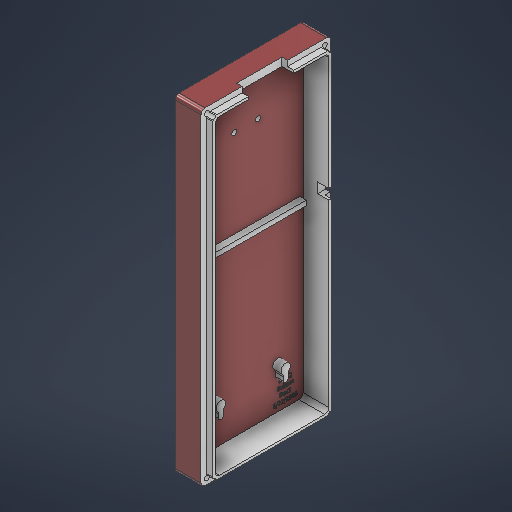
# Autodesk Inventor part: cDAQ_Bottom_Box3
Saved by Autodesk Inventor 2027 (Build 310192000, 192)
## iProperties
Created: 2026-05-08
Part Number: cDAQ_Bottom_Box3
Material: Generic
Document SubType Name: Modeling
Designer: giese
Density: 1 g/cm^3
Appearance: Default
Author: giese
Autodesk Inventor part; units mm, degrees
(part 1 of 2)
ref_plane "YZ Plane" through (0, 0, 0) normal (1, 0, 0) x (0, 1, 0)
ref_plane "XZ Plane" through (0, 0, 0) normal (0, 1, 0) x (-1, 0, 0)
ref_plane "XY Plane" through (0, 0, 0) normal (0, 0, 1) x (1, 0, 0)
sketch "Sketch1" plane through (0, 0, 0) normal (1, 0, 0) x (0, 1, 0)
  line L0 (37.5698, 53.1667) -> (-218.9702, 53.1667)
  line L1 (-218.9702, 53.1667) -> (-218.9702, -48.4333)
  line L2 (-218.9702, -48.4333) -> (37.5698, -48.4333)
  line L3 (37.5698, -48.4333) -> (37.5698, 53.1667)
  point P0 (0, 0)
  dimension "d0" = 101.6
  dimension "d1" = 256.54
  constraints: 8 end point, 2 parallel, 1 horizontal, 1 perpendicular
  measures "d0" distance of L2.end L0.start
  measures "d1" distance of L1.end L2.end
extrude "Extrusion1" add sketch "Sketch1" along normal blind 20.32
sketch "Sketch2" plane through (20.32, 0, 0) normal (1, 0, 0) x (0, 0, -1)
  line L0 (42.0833, 31.2198) -> (-46.8167, 31.2198)
  line L1 (-46.8167, 31.2198) -> (-46.8167, -212.6202)
  line L2 (-46.8167, -212.6202) -> (42.0833, -212.6202)
  line L3 (42.0833, -212.6202) -> (42.0833, 31.2198)
  line L4 (48.4333, 37.5698) -> (-53.1667, 37.5698) projected
  line L5 (-53.1667, 37.5698) -> (-53.1667, -218.9702) projected
  point P0 (0, 0)
  dimension "d4" = 243.84
  dimension "d5" = 88.9
  dimension "d8" = 6.35
  dimension "d21" = 6.35
  constraints: 8 end point, 2 parallel, 1 horizontal, 1 perpendicular
  measures "d4" distance of L2.end L0.start
  measures "d5" distance of L0.start L0.end
  measures "d8" distance between parallel lines of L0 L4
  measures "d21" distance between parallel lines of L5 L1
extrude "Extrusion2" cut sketch "Sketch2" against normal blind 15.24
sketch "Sketch3" plane through (0, 0, 0) normal (-1, 0, 0) x (0, 0, 1)
  circle A0 centre (-6.6909, -5.8642) radius 2
  circle A1 centre (11.8079, -5.8642) radius 2
  circle A2 centre (30.3067, -5.8642) radius 2
  line L0 (-48.4333, -218.9702) -> (-48.4333, 37.5698) projected
  line L1 (-48.4333, 37.5698) -> (53.1667, 37.5698) projected
  line L2 (53.1667, 37.5698) -> (53.1667, -218.9702) projected
  line L3 (46.8167, 31.2198) -> (-42.0833, 31.2198) projected
  point P0 (0, 0)
  point P1 (-0.896, -23.7433)
  point P2 (-45.1848, 27.0137)
  dimension "d9" = 18.4988
  dimension "d10" = 4
  dimension "d11" = 4
  dimension "d12" = 18.4988
  dimension "d13" = 36.9976
  dimension "d18" = 22.86
  dimension "d22" = 4
  dimension "d58" = 43.434
  constraints: 3 centre point
  measures "d9" distance of A0.centre A1.centre
  measures "d10" diameter of A1
  measures "d11" diameter of A2
  measures "d12" distance of A1.centre A2.centre
  measures "d13" distance of A0.centre A2.centre
  measures "d18" distance from line of L2 A2.centre
  measures "d22" diameter of A0
  measures "d58" distance from line of L1 A2.centre
extrude "Extrusion3" cut sketch "Sketch3" against normal blind 5.08
sketch "Sketch5" plane through (0, -218.9702, -48.4333) normal (0, 0, -1) x (-1, 0, 0)
  line L0 (-27.2034, 150.2918) -> (-16.51, 150.2918)
  line L1 (-16.51, 150.2918) -> (-16.51, 158.2918)
  line L2 (-16.51, 158.2918) -> (-27.2034, 158.2918)
  line L3 (-27.2034, 158.2918) -> (-27.2034, 150.2918)
  line L4 (0, 256.54) -> (-20.32, 256.54) projected
  line L5 (0, 0) -> (0, 256.54) projected
  line L6 (-20.32, 0) -> (-20.32, 256.54) projected
  point P0 (0, 218.9702)
  point P1 (-21.8567, 158.2918)
  point P2 (-21.8567, 150.2918)
  dimension "d28" = 10.6934
  dimension "d30" = 8
  dimension "d31" = 16.51
  dimension "d34" = 106.2482
  dimension "d215" = 6.8834
  constraints: 8 end point, 2 midpoint, 2 parallel, 1 horizontal, 1 perpendicular
  measures "d28" distance between parallel lines of L1 L3
  measures "d30" distance of point (-21.857, 158.292) point (-21.857, 150.292)
  measures "d31" distance between parallel lines of L5 L1
  measures "d34" distance between parallel lines of L4 L0
  measures "d215" distance between parallel lines of L6 L3
extrude "Extrusion4" cut sketch "Sketch5" against normal blind 24.13
sketch "Sketch6" plane through (0, -218.9702, -48.4333) normal (0, -1, 0) x (1, 0, 0)
  line L0 (24.08, 45.1284) -> (16.08, 45.1284)
  line L1 (16.08, 45.1284) -> (16.08, 35.1284)
  line L2 (16.08, 35.1284) -> (24.08, 35.1284)
  line L3 (0, 101.6) -> (0, 0) projected
  line L4 (25.82, 43.1283) -> (25.82, 37.1284)
  line L5 (24.08, 45.1284) -> (25.82, 43.1283)
  line L6 (25.82, 37.1284) -> (24.08, 35.1284)
  line L7 (0, 0) -> (20.32, 0) projected
  line L8 (20.32, 95.25) -> (20.32, 6.35) projected
  line L9 (20.32, 41.9134) -> (20.32, 37.4697)
  point P0 (0, 48.4333)
  point P1 (20.08, 45.1284)
  point P2 (20.08, 35.1284)
  point P3 (16.08, 40.1284)
  dimension "d35" = 10
  dimension "d39" = 6
  dimension "d48" = 45.1284
  dimension "d220" = 16.08
  dimension "d221" = 0
  dimension "d222" = 8
  dimension "d223" = 2
  dimension "d224" = 2
  dimension "d225" = 5.5
  dimension "d226" = 4.24
  dimension "d227" = 1.74
  constraints: 14 end point, 3 midpoint, 2 point on line, 1 horizontal, 1 parallel, 1 perpendicular, 1 vertical
  measures "d35" distance of point (20.08, 45.128) point (20.08, 35.128)
  measures "d39" distance of L4.start L4.end
  measures "d48" distance between parallel lines of L7 L0
  measures "d220" distance from line of L3 point (16.08, 40.128)
  measures "d221" horizontal distance of L0.start L2.end
  measures "d222" distance of L1.end L2.end
  measures "d223" vertical distance of L4.end L2.end
  measures "d224" vertical distance of L0.start L4.start
  measures "d225" distance between parallel lines of L4 L8
  measures "d226" distance between parallel lines of L1 L8
  measures "d227" distance from line of L2.end L4
extrude "Extrusion5" cut sketch "Sketch6" against normal blind 3.81
sketch "Sketch7" plane through (0, 37.5698, 53.1667) normal (0, 1, 0) x (1, 0, 0)
  line L0 (31.0134, 67.818) -> (16.002, 67.818)
  line L1 (16.002, 67.818) -> (16.002, 32.258)
  line L2 (16.002, 32.258) -> (31.0134, 32.258)
  line L3 (31.0134, 32.258) -> (31.0134, 67.818)
  line L4 (0, 0) -> (20.32, 0) projected
  line L5 (0, 101.6) -> (0, 0) projected
  line L6 (20.32, 101.6) -> (20.32, 0) projected
  point P0 (0, 53.1667)
  point P1 (20.32, 67.818)
  point P2 (20.32, 32.258)
  dimension "d51" = 35.56
  dimension "d52" = 32.258
  dimension "d55" = 16.002
  dimension "d56" = 15.0114
  dimension "d57" = 10.6934
  constraints: 8 end point, 2 parallel, 1 horizontal, 1 perpendicular
  measures "d51" distance of L2.end L0.start
  measures "d52" distance between parallel lines of L4 L2
  measures "d55" distance between parallel lines of L5 L1
  measures "d56" distance between parallel lines of L3 L1
  measures "d57" distance between parallel lines of L6 L3
extrude "Extrusion6" cut sketch "Sketch7" against normal blind 7.62
fillet "Fillet1" radius 3.175 4 edges at (10.16, 37.5698, -48.4333) (10.16, 37.5698, 53.1667) (10.16, -218.9702, -48.4333) (10.16, -218.9702, 53.1667)
sketch "Sketch8" plane through (0, 0, 0) normal (-1, 0, 0) x (0, 0, 1)
  line L0 (-8.4625, -9.3948) -> (-4.9319, -9.3948)
  line L1 (-8.4625, -2.3336) -> (-4.9319, -2.3336)
  line L2 (-8.4625, -9.3948) -> (-10.5009, -5.8642)
  line L3 (-8.4625, -2.3336) -> (-10.5009, -5.8642)
  line L4 (-4.9319, -9.3948) -> (-2.8936, -5.8642)
  line L5 (-4.9319, -2.3336) -> (-2.8936, -5.8642)
  circle A0 centre (-6.6909, -5.8642) radius 2 projected
  line L6 (10.0363, -9.3948) -> (13.5669, -9.3948)
  line L7 (10.0363, -2.3336) -> (13.5669, -2.3336)
  line L8 (10.0363, -9.3948) -> (7.9979, -5.8642)
  line L9 (10.0363, -2.3336) -> (7.9979, -5.8642)
  line L10 (13.5669, -9.3948) -> (15.6053, -5.8642)
  line L11 (13.5669, -2.3336) -> (15.6053, -5.8642)
  circle A1 centre (11.8079, -5.8642) radius 2 projected
  line L12 (28.5351, -9.3948) -> (26.4967, -5.8642)
  line L13 (28.5351, -2.3336) -> (26.4967, -5.8642)
  line L14 (28.5351, -9.3948) -> (32.0657, -9.3948)
  line L15 (28.5351, -2.3336) -> (32.0657, -2.3336)
  line L16 (32.0657, -9.3948) -> (34.1041, -5.8642)
  line L17 (32.0657, -2.3336) -> (34.1041, -5.8642)
  circle A2 centre (30.3067, -5.8642) radius 2 projected
  point P0 (-6.6972, -9.3948)
  point P1 (11.8016, -9.3948)
  point P2 (30.3004, -9.3948)
  point P3 (-10.5009, -5.8642)
  point P4 (-2.8936, -5.8642)
  point P5 (15.6053, -5.8642)
  point P6 (7.9979, -5.8642)
  point P7 (34.1041, -5.8642)
  dimension "d60" = 7.0612
  dimension "d61" = 120
  dimension "d62" = 120
  dimension "d63" = 120
  dimension "d64" = 120
  dimension "d65" = 3.5306
  dimension "d66" = 3.5306
  dimension "d67" = 3.5306
  dimension "d68" = 3.5306
  dimension "d69" = 3.5306
  dimension "d70" = 3.5306
  dimension "d71" = 0
  dimension "d72" = 7.6074
  dimension "d73" = 3.81
  dimension "d74" = 0
  dimension "d75" = 7.0612
  dimension "d76" = 120
  dimension "d77" = 120
  dimension "d78" = 120
  dimension "d79" = 120
  dimension "d80" = 3.5306
  dimension "d81" = 3.5306
  dimension "d82" = 3.5306
  dimension "d83" = 3.5306
  dimension "d84" = 3.5306
  dimension "d85" = 3.5306
  dimension "d86" = 0
  dimension "d87" = 7.6074
  dimension "d91" = 0
  dimension "d92" = 3.81
  dimension "d93" = 7.0612
  dimension "d94" = 120
  dimension "d95" = 120
  dimension "d96" = 120
  dimension "d97" = 120
  dimension "d98" = 3.5306
  dimension "d99" = 3.5306
  dimension "d100" = 3.5306
  dimension "d101" = 3.5306
  dimension "d102" = 3.5306
  dimension "d103" = 3.5306
  dimension "d104" = 0
  dimension "d105" = 7.6074
  dimension "d108" = 0
  dimension "d109" = 3.81
  constraints: 36 end point, 6 horizontal, 3 midpoint
  measures "d60" distance from line of point (-6.697, -9.395) L1
  measures "d61" angle of L0 L2
  measures "d62" angle of L1 L3
  measures "d63" angle of L4 L0
  measures "d64" angle of L5 L1
  measures "d65" distance of L0.start L0.end
  measures "d66" distance of L1.start L1.end
  measures "d67" vertical distance of L1.start L3.end
  measures "d68" vertical distance of L0.start L2.end
  measures "d69" vertical distance of L1.end L5.end
  measures "d70" vertical distance of L0.end L4.end
  measures "d71" horizontal distance of L0.start L1.start
  measures "d72" distance of L4.end L2.end
  measures "d73" distance of A0.centre L2.end
  measures "d74" vertical distance of A0.centre L4.end
  measures "d75" distance from line of point (11.802, -9.395) L7
  measures "d76" angle of L6 L8
  measures "d77" angle of L7 L9
  measures "d78" angle of L10 L6
  measures "d79" angle of L11 L7
  measures "d80" distance of L8.start L6.end
  measures "d81" distance of L9.start L7.end
  measures "d82" vertical distance of L9.start L9.end
  measures "d83" vertical distance of L8.start L8.end
  measures "d84" vertical distance of L7.end L11.end
  measures "d85" vertical distance of L6.end L10.end
  measures "d86" horizontal distance of L8.start L9.start
  measures "d87" distance of L10.end L8.end
  measures "d91" vertical distance of A1.centre L8.end
  measures "d92" distance of A1.centre L8.end
  measures "d93" distance from line of point (30.3, -9.395) L15
  measures "d94" angle of L14 L12
  measures "d95" angle of L15 L13
  measures "d96" angle of L16 L14
  measures "d97" angle of L17 L15
  measures "d98" distance of L12.start L16.start
  measures "d99" distance of L15.start L15.end
  measures "d100" vertical distance of L15.start L13.end
  measures "d101" vertical distance of L12.start L12.end
  measures "d102" vertical distance of L15.end L17.end
  measures "d103" vertical distance of L16.start L16.end
  measures "d104" horizontal distance of L12.start L15.start
  measures "d105" distance of L16.end L12.end
  measures "d108" vertical distance of A2.centre L12.end
  measures "d109" distance of A2.centre L12.end
extrude "Extrusion7" cut sketch "Sketch8" against normal blind 0.9525 contours L2 L3 L1 L5 L4 L0 | A0 | L8 L9 L7 L11 L10 L6 | A1 | L12 L13 L15 L17 L16 L14 | A2
sketch "Sketch9" plane through (5.08, 0, 0) normal (1, 0, 0) x (0, 0, -1)
  arc A0 (24.8089, -182.3284) -> (19.3527, -182.3284) centre (22.0808, -179.8542) ccw
  line L0 (45.2583, 37.5698) -> (14.6513, 37.5698) projected
  line L1 (42.0833, 31.2198) -> (42.0833, -212.6202) projected
  arc A1 (20.1758, -187.4742) -> (23.9858, -187.4742) centre (22.0808, -187.4742) ccw
  line L2 (23.9858, -187.4742) -> (23.9858, -184.4614)
  line L3 (20.1758, -187.4742) -> (20.1758, -184.4614)
  arc A2 (24.8089, -182.3284) -> (23.9858, -184.4614) centre (27.1608, -184.4614) ccw
  arc A3 (20.1758, -184.4614) -> (19.3527, -182.3284) centre (17.0008, -184.4614) ccw
  arc A4 (-25.9911, -182.3284) -> (-31.4473, -182.3285) centre (-28.7192, -179.8542) ccw
  arc A5 (-30.6242, -187.4606) -> (-26.8142, -187.4742) centre (-28.7192, -187.4742) ccw
  line L4 (-26.8142, -187.4742) -> (-26.8142, -184.4614)
  line L5 (-30.6242, -187.4606) -> (-30.6242, -184.4614)
  arc A6 (-25.9911, -182.3284) -> (-26.8142, -184.4614) centre (-23.6392, -184.4614) ccw
  arc A7 (-30.6242, -184.4614) -> (-31.4473, -182.3285) centre (-33.7992, -184.4614) ccw
  line L6 (-20.9087, 37.5698) -> (-49.9917, 37.5698) projected
  line L7 (-46.8167, -212.6202) -> (-46.8167, 31.2198) projected
  point P0 (0, 0)
  point P1 (23.9858, -183.0063)
  point P2 (20.1758, -183.0063)
  point P3 (-26.8142, -183.0063)
  point P4 (-30.6242, -183.0063)
  dimension "d112" = 217.424
  dimension "d114" = 7.366
  dimension "d116" = 3.81
  dimension "d117" = 225.044
  dimension "d118" = 3.175
  dimension "d119" = 7.366
  dimension "d120" = 3.81
  dimension "d121" = 3.175
  dimension "d122" = 217.424
  dimension "d123" = 225.044
  dimension "d125" = 0
  dimension "d128" = 50.8
  dimension "d129" = 20.0025
  dimension "d130" = 0
  constraints: 20 point on circle, 8 centre point, 8 end point, 8 tangent, 4 point on line, 2 equal radius, 2 parallel, 2 vertical
  measures "d112" distance from line of L0 A0.centre
  measures "d114" diameter of A0
  measures "d116" diameter of A1
  measures "d117" distance from line of L0 A1.centre
  measures "d118" radius of A2
  measures "d119" diameter of A4
  measures "d120" diameter of A5
  measures "d121" radius of A6
  measures "d122" distance from line of A4.centre L6
  measures "d123" distance from line of L6 A5.centre
  measures "d125" horizontal distance of A5.centre A4.centre
  measures "d128" distance of A5.centre A1.centre
  measures "d129" distance from line of L1 A0.centre
  measures "d130" horizontal distance of A0.centre A1.centre
extrude "Extrusion8" add sketch "Sketch9" along normal blind 6.4008
sketch "Sketch10" plane through (20.32, 0, 0) normal (1, 0, 0) x (0, 0, -1)
  line L0 (-46.8167, 31.2198) -> (42.0833, 31.2198) projected
  line L1 (-46.8167, 31.2198) -> (42.0833, 31.2198)
  line L2 (42.0833, 33.2264) -> (-46.8167, 33.2264)
  line L3 (-46.8167, 33.2264) -> (-48.8233, 33.2264)
  line L4 (-48.8233, 33.2264) -> (-48.8233, -214.6268)
  line L5 (-48.8233, -214.6268) -> (44.0899, -214.6268)
  line L6 (44.0899, -214.6268) -> (44.0899, 33.2264)
  line L7 (44.0899, 33.2264) -> (41.9392, 33.2264)
  line L8 (42.0833, 31.2198) -> (42.0833, -212.6202) projected
  line L9 (-46.8167, -212.6202) -> (-46.8167, 31.2198) projected
  line L10 (42.0833, -212.6202) -> (-46.8167, -212.6202) projected
  line L11 (45.2583, 37.5698) -> (14.6513, 37.5698) projected
  dimension "d202" = 2.0066
  dimension "d203" = 2.0066
  dimension "d204" = 2.0066
  dimension "d205" = 2.0066
  dimension "d208" = 4.3434
  constraints: 14 end point, 3 perpendicular, 3 point on line, 1 collinear, 1 horizontal
  measures "d202" distance between parallel lines of L0 L2
  measures "d203" distance between parallel lines of L6 L8
  measures "d204" distance between parallel lines of L4 L9
  measures "d205" distance between parallel lines of L5 L10
  measures "d208" distance between parallel lines of L11 L2
extrude "Extrusion9" add sketch "Sketch10" along normal blind 5
fillet "Fillet2" radius 3.175 8 edges at (15.2, 31.2198, -42.0833) (15.2, 31.2198, 46.8167) (15.2, -212.6202, 46.8167) (15.2, -212.6202, -42.0833) (22.82, 33.2264, -44.0899) (22.82, 33.2264, 48.8233) (22.82, -214.6268, -44.0899) (22.82, -214.6268, 48.8233)
sketch "Sketch13" plane through (25.32, 0, 0) normal (1, 0, 0) x (0, 0, -1)
  arc A0 (44.0833, 30.0448) -> (40.9083, 33.2198) centre (40.9083, 30.0448) ccw projected
  arc A1 (-45.6417, 33.2198) -> (-48.8167, 30.0448) centre (-45.6417, 30.0448) ccw projected
  arc A2 (40.9083, -212.0802) -> (44.0833, -208.9052) centre (40.9083, -208.9052) ccw projected
  arc A3 (-48.8167, -208.9052) -> (-45.6417, -212.0802) centre (-45.6417, -208.9052) ccw projected
  line L0 (-20.9087, 37.5698) -> (-49.9917, 37.5698) projected
  line L1 (-53.1667, 34.3948) -> (-53.1667, -215.7952) projected
  line L2 (-49.9917, -218.9702) -> (45.2583, -218.9702) projected
  arc A4 (-48.8167, -208.9052) -> (-45.6417, -212.0802) centre (-45.6417, -208.9052) ccw projected
  circle A5 centre (-48.5947, -214.3982) radius 1.9939
  circle A6 centre (43.8613, -214.3982) radius 1.9939
  line L3 (48.4333, -215.7952) -> (48.4333, 34.3948) projected
  circle A7 centre (43.8613, 32.9978) radius 1.9939
  line L4 (45.2583, 37.5698) -> (14.6513, 37.5698) projected
  circle A8 centre (-48.5947, 32.9978) radius 1.9939
  point P0 (0, 0)
  point P1 (-47.8868, 32.2898)
  point P2 (-47.8868, -211.1503)
  point P3 (-47.8868, -211.1503)
  dimension "d178" = 4.572
  dimension "d179" = 4.572
  dimension "d180" = 3.9878
  dimension "d181" = 4.572
  dimension "d182" = 4.572
  dimension "d183" = 3.9878
  dimension "d184" = 3.9878
  dimension "d185" = 4.572
  dimension "d186" = 4.572
  dimension "d187" = 3.9878
  dimension "d188" = 4.572
  dimension "d189" = 4.572
  constraints: 4 centre point, 3 point on circle
  measures "d178" distance from line of L1 A5.centre
  measures "d179" distance from line of L2 A5.centre
  measures "d180" diameter of A5
  measures "d181" distance from line of L2 A6.centre
  measures "d182" distance from line of L3 A6.centre
  measures "d183" diameter of A6
  measures "d184" diameter of A7
  measures "d185" distance from line of L3 A7.centre
  measures "d186" distance from line of L4 A7.centre
  measures "d187" diameter of A8
  measures "d188" distance from line of L0 A8.centre
  measures "d189" distance from line of L1 A8.centre
extrude "Extrusion11" cut sketch "Sketch13" against normal blind 25.4
sketch "Sketch14" plane through (5.08, 0, 0) normal (1, 0, 0) x (0, 0, -1)
  line L0 (18.5513, -190.7882) -> (37.7681, -190.7882) construction
  line L1 (37.7681, -190.7882) -> (37.7681, -199.5809) construction
  line L2 (37.7681, -199.5809) -> (18.5513, -199.5809) construction
  line L3 (18.5513, -199.5809) -> (18.5513, -190.7882) construction
  spline S0 degree 2 poles (24.2188, -193.9523) (23.9817, -193.9523) (23.5889, -193.8066) (23.4481, -193.6584) knots 0 0 0 1 2 2 2
  spline S1 degree 2 poles (23.4481, -193.6584) (23.3073, -193.5127) (23.1517, -193.0631) (23.1517, -192.7618) knots 0 0 0 1 2 2 2
  spline S2 degree 2 poles (23.1517, -192.7618) (23.1517, -192.4604) (23.3123, -192.0208) (23.4481, -191.8726) knots 0 0 0 1 2 2 2
  spline S3 degree 2 poles (23.4481, -191.8726) (23.584, -191.7219) (23.9866, -191.5614) (24.2188, -191.5614) knots 0 0 0 1 2 2 2
  spline S4 degree 2 poles (24.2188, -191.5614) (24.4065, -191.5614) (24.7572, -191.6676) (24.8931, -191.7367) knots 0 0 0 1 2 2 2
  line L4 (24.8931, -191.7367) -> (24.8931, -192.169)
  line L5 (24.8931, -192.169) -> (24.8709, -192.169)
  spline S5 degree 2 poles (24.8709, -192.169) (24.8289, -192.1344) (24.7004, -192.0455) (24.609, -191.9985) knots 0 0 0 1 2 2 2
  spline S6 degree 2 poles (24.609, -191.9985) (24.5275, -191.959) (24.3102, -191.8973) (24.2114, -191.8973) knots 0 0 0 1 2 2 2
  spline S7 degree 2 poles (24.2114, -191.8973) (23.9125, -191.8973) (23.5494, -192.3493) (23.5494, -192.7618) knots 0 0 0 1 2 2 2
  spline S8 degree 2 poles (23.5494, -192.7618) (23.5494, -193.1644) (23.9002, -193.6164) (24.2114, -193.6164) knots 0 0 0 1 2 2 2
  spline S9 degree 2 poles (24.2114, -193.6164) (24.3991, -193.6164) (24.74, -193.4608) (24.8709, -193.3398) knots 0 0 0 1 2 2 2
  line L6 (24.8709, -193.3398) -> (24.8931, -193.3398)
  line L7 (24.8931, -193.3398) -> (24.8931, -193.772)
  spline S10 degree 2 poles (24.8931, -193.772) (24.8363, -193.7992) (24.6634, -193.8758) (24.5942, -193.8931) knots 0 0 0 1 2 2 2
  spline S11 degree 2 poles (24.5942, -193.8931) (24.4954, -193.9227) (24.3398, -193.9523) (24.2188, -193.9523) knots 0 0 0 1 2 2 2
  spline S12 degree 2 poles (27.6768, -192.3789) (27.6768, -192.7964) (27.3384, -193.4682) (27.0544, -193.6559) knots 0 0 0 1 2 2 2
  spline S13 degree 2 poles (27.0544, -193.6559) (26.8222, -193.8017) (26.3455, -193.9005) (25.975, -193.9005) knots 0 0 0 1 2 2 2
  line L8 (25.975, -193.9005) -> (25.2735, -193.9005)
  line L9 (25.2735, -193.9005) -> (25.2735, -190.8525)
  line L10 (25.2735, -190.8525) -> (25.9676, -190.8525)
  spline S14 degree 2 poles (25.9676, -190.8525) (26.3973, -190.8525) (26.8864, -190.9809) (27.0593, -191.0945) knots 0 0 0 1 2 2 2
  spline S15 degree 2 poles (27.0593, -191.0945) (27.3532, -191.2897) (27.6768, -191.9343) (27.6768, -192.3789) knots 0 0 0 1 2 2 2
  spline S16 degree 2 poles (27.2544, -192.374) (27.2544, -192.0233) (27.0223, -191.5268) (26.7925, -191.386) knots 0 0 0 1 2 2 2
  spline S17 degree 2 poles (26.7925, -191.386) (26.6295, -191.2897) (26.2615, -191.2032) (25.9873, -191.2032) knots 0 0 0 1 2 2 2
  line L11 (25.9873, -191.2032) -> (25.6786, -191.2032)
  line L12 (25.6786, -191.2032) -> (25.6786, -193.5497)
  line L13 (25.6786, -193.5497) -> (25.9873, -193.5497)
  spline S18 degree 2 poles (25.9873, -193.5497) (26.2565, -193.5497) (26.6641, -193.4633) (26.8296, -193.3472) knots 0 0 0 1 2 2 2
  spline S19 degree 2 poles (26.8296, -193.3472) (27.042, -193.2039) (27.2544, -192.7297) (27.2544, -192.374) knots 0 0 0 1 2 2 2
  line L14 (27.788, -193.9005) -> (28.8155, -190.8525)
  line L15 (28.8155, -190.8525) -> (29.3144, -190.8525)
  line L16 (29.3144, -190.8525) -> (30.342, -193.9005)
  line L17 (30.342, -193.9005) -> (29.9146, -193.9005)
  line L18 (29.9146, -193.9005) -> (29.638, -193.0483)
  line L19 (29.638, -193.0483) -> (28.4746, -193.0483)
  line L20 (28.4746, -193.0483) -> (28.198, -193.9005)
  line L21 (28.198, -193.9005) -> (27.788, -193.9005)
  line L22 (29.5268, -192.7025) -> (29.0551, -191.2674)
  line L23 (29.0551, -191.2674) -> (28.5858, -192.7025)
  line L24 (28.5858, -192.7025) -> (29.5268, -192.7025)
  spline S20 degree 2 poles (33.1627, -194.6464) (33.0516, -194.6736) (32.8095, -194.7032) (32.6885, -194.7032) knots 0 0 0 1 2 2 2
  spline S21 degree 2 poles (32.6885, -194.7032) (32.3451, -194.7032) (31.9178, -194.3204) (31.8981, -193.9647) knots 0 0 0 1 2 2 2
  spline S22 degree 2 poles (31.8981, -193.9647) (31.8709, -193.9647) (31.824, -193.9647) (31.8042, -193.9647) knots 0 0 0 1 2 2 2
  spline S23 degree 2 poles (31.8042, -193.9647) (31.4955, -193.9647) (30.999, -193.7547) (30.8211, -193.5497) knots 0 0 0 1 2 2 2
  spline S24 degree 2 poles (30.8211, -193.5497) (30.6458, -193.3472) (30.458, -192.7544) (30.458, -192.3789) knots 0 0 0 1 2 2 2
  spline S25 degree 2 poles (30.458, -192.3789) (30.458, -191.9936) (30.6482, -191.4107) (30.8236, -191.2032) knots 0 0 0 1 2 2 2
  spline S26 degree 2 poles (30.8236, -191.2032) (31.0014, -190.9982) (31.4979, -190.7882) (31.8042, -190.7882) knots 0 0 0 1 2 2 2
  spline S27 degree 2 poles (31.8042, -190.7882) (32.1154, -190.7882) (32.6144, -191.0056) (32.7873, -191.2032) knots 0 0 0 1 2 2 2
  spline S28 degree 2 poles (32.7873, -191.2032) (32.9602, -191.4033) (33.1528, -191.9985) (33.1528, -192.3789) knots 0 0 0 1 2 2 2
  spline S29 degree 2 poles (33.1528, -192.3789) (33.1528, -192.9717) (32.6909, -193.7424) (32.2883, -193.8782) knots 0 0 0 1 2 2 2
  spline S30 degree 2 poles (32.2883, -193.8782) (32.2982, -193.9919) (32.3575, -194.1746) (32.4044, -194.2265) knots 0 0 0 1 2 2 2
  spline S31 degree 2 poles (32.4044, -194.2265) (32.4612, -194.2907) (32.6168, -194.35) (32.7552, -194.35) knots 0 0 0 1 2 2 2
  spline S32 degree 2 poles (32.7552, -194.35) (32.8367, -194.35) (33.059, -194.2981) (33.1084, -194.2784) knots 0 0 0 1 2 2 2
  line L25 (33.1084, -194.2784) -> (33.1627, -194.2784)
  line L26 (33.1627, -194.2784) -> (33.1627, -194.6464)
  spline S33 degree 2 poles (32.7305, -192.3789) (32.7305, -192.0751) (32.5995, -191.6083) (32.481, -191.4551) knots 0 0 0 1 2 2 2
  spline S34 degree 2 poles (32.481, -191.4551) (32.36, -191.2971) (32.0191, -191.139) (31.8067, -191.139) knots 0 0 0 1 2 2 2
  spline S35 degree 2 poles (31.8067, -191.139) (31.5868, -191.139) (31.2559, -191.2921) (31.1299, -191.4551) knots 0 0 0 1 2 2 2
  spline S36 degree 2 poles (31.1299, -191.4551) (31.0089, -191.6108) (30.8804, -192.0825) (30.8804, -192.3789) knots 0 0 0 1 2 2 2
  spline S37 degree 2 poles (30.8804, -192.3789) (30.8804, -192.9791) (31.3843, -193.6189) (31.8067, -193.6189) knots 0 0 0 1 2 2 2
  spline S38 degree 2 poles (31.8067, -193.6189) (32.229, -193.6189) (32.7305, -192.9791) (32.7305, -192.3789) knots 0 0 0 1 2 2 2
  spline S39 degree 2 poles (23.8631, -197.9828) (23.8631, -198.21) (23.6902, -198.5583) (23.5469, -198.6719) knots 0 0 0 1 2 2 2
  spline S40 degree 2 poles (23.5469, -198.6719) (23.374, -198.8053) (22.9813, -198.9189) (22.6701, -198.9189) knots 0 0 0 1 2 2 2
  line L27 (22.6701, -198.9189) -> (21.7957, -198.9189)
  line L28 (21.7957, -198.9189) -> (21.7957, -195.8709)
  line L29 (21.7957, -195.8709) -> (22.6034, -195.8709)
  spline S41 degree 2 poles (22.6034, -195.8709) (22.9294, -195.8709) (23.2555, -195.9129) (23.4037, -195.9944) knots 0 0 0 1 2 2 2
  spline S42 degree 2 poles (23.4037, -195.9944) (23.5692, -196.0809) (23.7198, -196.3649) (23.7198, -196.5576) knots 0 0 0 1 2 2 2
  spline S43 degree 2 poles (23.7198, -196.5576) (23.7198, -196.7725) (23.4926, -197.1133) (23.2925, -197.2097) knots 0 0 0 1 2 2 2
  line L30 (23.2925, -197.2097) -> (23.2925, -197.2245)
  spline S44 degree 2 poles (23.2925, -197.2245) (23.5642, -197.2986) (23.8631, -197.6913) (23.8631, -197.9828) knots 0 0 0 1 2 2 2
  spline S45 degree 2 poles (23.4407, -198.0001) (23.4407, -197.8272) (23.3419, -197.6049) (23.1937, -197.5258) knots 0 0 0 1 2 2 2
  spline S46 degree 2 poles (23.1937, -197.5258) (23.0974, -197.4764) (22.8702, -197.4468) (22.6602, -197.4468) knots 0 0 0 1 2 2 2
  line L31 (22.6602, -197.4468) -> (22.2008, -197.4468)
  line L32 (22.2008, -197.4468) -> (22.2008, -198.5731)
  line L33 (22.2008, -198.5731) -> (22.5293, -198.5731)
  spline S47 degree 2 poles (22.5293, -198.5731) (22.7961, -198.5731) (23.1023, -198.5237) (23.2209, -198.4447) knots 0 0 0 1 2 2 2
  spline S48 degree 2 poles (23.2209, -198.4447) (23.3345, -198.3632) (23.4407, -198.1606) (23.4407, -198.0001) knots 0 0 0 1 2 2 2
  spline S49 degree 2 poles (23.2975, -196.6144) (23.2975, -196.5057) (23.2234, -196.3427) (23.1419, -196.2958) knots 0 0 0 1 2 2 2
  spline S50 degree 2 poles (23.1419, -196.2958) (23.0431, -196.2414) (22.8035, -196.2167) (22.5886, -196.2167) knots 0 0 0 1 2 2 2
  line L34 (22.5886, -196.2167) -> (22.2008, -196.2167)
  line L35 (22.2008, -196.2167) -> (22.2008, -197.1084)
  line L36 (22.2008, -197.1084) -> (22.6602, -197.1084)
  spline S51 degree 2 poles (22.6602, -197.1084) (22.8504, -197.1084) (23.0307, -197.0689) (23.127, -197.0071) knots 0 0 0 1 2 2 2
  spline S52 degree 2 poles (23.127, -197.0071) (23.2209, -196.9478) (23.2975, -196.7576) (23.2975, -196.6144) knots 0 0 0 1 2 2 2
  spline S53 degree 2 poles (26.1158, -197.7753) (26.1158, -198.3533) (25.56, -198.9831) (25.0956, -198.9831) knots 0 0 0 1 2 2 2
  spline S54 degree 2 poles (25.0956, -198.9831) (24.6189, -198.9831) (24.0731, -198.3335) (24.0731, -197.7753) knots 0 0 0 1 2 2 2
  spline S55 degree 2 poles (24.0731, -197.7753) (24.0731, -197.2023) (24.6362, -196.5675) (25.0956, -196.5675) knots 0 0 0 1 2 2 2
  spline S56 degree 2 poles (25.0956, -196.5675) (25.56, -196.5675) (26.1158, -197.1998) (26.1158, -197.7753) knots 0 0 0 1 2 2 2
  spline S57 degree 2 poles (25.7181, -197.7753) (25.7181, -197.3307) (25.3945, -196.8984) (25.0956, -196.8984) knots 0 0 0 1 2 2 2
  spline S58 degree 2 poles (25.0956, -196.8984) (24.7968, -196.8984) (24.4707, -197.3307) (24.4707, -197.7753) knots 0 0 0 1 2 2 2
  spline S59 degree 2 poles (24.4707, -197.7753) (24.4707, -198.2075) (24.7968, -198.6522) (25.0956, -198.6522) knots 0 0 0 1 2 2 2
  spline S60 degree 2 poles (25.0956, -198.6522) (25.392, -198.6522) (25.7181, -198.215) (25.7181, -197.7753) knots 0 0 0 1 2 2 2
  spline S61 degree 2 poles (27.2026, -198.9634) (26.8889, -198.9634) (26.5357, -198.6052) (26.5357, -198.2174) knots 0 0 0 1 2 2 2
  line L37 (26.5357, -198.2174) -> (26.5357, -196.9503)
  line L38 (26.5357, -196.9503) -> (26.2763, -196.9503)
  line L39 (26.2763, -196.9503) -> (26.2763, -196.6317)
  line L40 (26.2763, -196.6317) -> (26.5357, -196.6317)
  line L41 (26.5357, -196.6317) -> (26.5357, -195.9747)
  line L42 (26.5357, -195.9747) -> (26.921, -195.9747)
  line L43 (26.921, -195.9747) -> (26.921, -196.6317)
  line L44 (26.921, -196.6317) -> (27.6299, -196.6317)
  line L45 (27.6299, -196.6317) -> (27.6299, -196.9503)
  line L46 (27.6299, -196.9503) -> (26.921, -196.9503)
  line L47 (26.921, -196.9503) -> (26.921, -198.0396)
  spline S62 degree 2 poles (26.921, -198.0396) (26.921, -198.2125) (26.9333, -198.4027) (26.9753, -198.4842) knots 0 0 0 1 2 2 2
  spline S63 degree 2 poles (26.9753, -198.4842) (27.0099, -198.5558) (27.1655, -198.6275) (27.2989, -198.6275) knots 0 0 0 1 2 2 2
  spline S64 degree 2 poles (27.2989, -198.6275) (27.3928, -198.6275) (27.5681, -198.5706) (27.6076, -198.5534) knots 0 0 0 1 2 2 2
  line L48 (27.6076, -198.5534) -> (27.6299, -198.5534)
  line L49 (27.6299, -198.5534) -> (27.6299, -198.8992)
  spline S65 degree 2 poles (27.6299, -198.8992) (27.5212, -198.9288) (27.2989, -198.9634) (27.2026, -198.9634) knots 0 0 0 1 2 2 2
  spline S66 degree 2 poles (28.6055, -198.9634) (28.2918, -198.9634) (27.9386, -198.6052) (27.9386, -198.2174) knots 0 0 0 1 2 2 2
  line L50 (27.9386, -198.2174) -> (27.9386, -196.9503)
  line L51 (27.9386, -196.9503) -> (27.6793, -196.9503)
  line L52 (27.6793, -196.9503) -> (27.6793, -196.6317)
  line L53 (27.6793, -196.6317) -> (27.9386, -196.6317)
  line L54 (27.9386, -196.6317) -> (27.9386, -195.9747)
  line L55 (27.9386, -195.9747) -> (28.324, -195.9747)
  line L56 (28.324, -195.9747) -> (28.324, -196.6317)
  line L57 (28.324, -196.6317) -> (29.0328, -196.6317)
  line L58 (29.0328, -196.6317) -> (29.0328, -196.9503)
  line L59 (29.0328, -196.9503) -> (28.324, -196.9503)
  line L60 (28.324, -196.9503) -> (28.324, -198.0396)
  spline S67 degree 2 poles (28.324, -198.0396) (28.324, -198.2125) (28.3363, -198.4027) (28.3783, -198.4842) knots 0 0 0 1 2 2 2
  spline S68 degree 2 poles (28.3783, -198.4842) (28.4129, -198.5558) (28.5685, -198.6275) (28.7019, -198.6275) knots 0 0 0 1 2 2 2
  spline S69 degree 2 poles (28.7019, -198.6275) (28.7957, -198.6275) (28.9711, -198.5706) (29.0106, -198.5534) knots 0 0 0 1 2 2 2
  line L61 (29.0106, -198.5534) -> (29.0328, -198.5534)
  line L62 (29.0328, -198.5534) -> (29.0328, -198.8992)
  spline S70 degree 2 poles (29.0328, -198.8992) (28.9242, -198.9288) (28.7019, -198.9634) (28.6055, -198.9634) knots 0 0 0 1 2 2 2
  spline S71 degree 2 poles (31.1966, -197.7753) (31.1966, -198.3533) (30.6408, -198.9831) (30.1765, -198.9831) knots 0 0 0 1 2 2 2
  spline S72 degree 2 poles (30.1765, -198.9831) (29.6998, -198.9831) (29.1539, -198.3335) (29.1539, -197.7753) knots 0 0 0 1 2 2 2
  spline S73 degree 2 poles (29.1539, -197.7753) (29.1539, -197.2023) (29.717, -196.5675) (30.1765, -196.5675) knots 0 0 0 1 2 2 2
  spline S74 degree 2 poles (30.1765, -196.5675) (30.6408, -196.5675) (31.1966, -197.1998) (31.1966, -197.7753) knots 0 0 0 1 2 2 2
  spline S75 degree 2 poles (30.7989, -197.7753) (30.7989, -197.3307) (30.4753, -196.8984) (30.1765, -196.8984) knots 0 0 0 1 2 2 2
  spline S76 degree 2 poles (30.1765, -196.8984) (29.8776, -196.8984) (29.5515, -197.3307) (29.5515, -197.7753) knots 0 0 0 1 2 2 2
  spline S77 degree 2 poles (29.5515, -197.7753) (29.5515, -198.2075) (29.8776, -198.6522) (30.1765, -198.6522) knots 0 0 0 1 2 2 2
  spline S78 degree 2 poles (30.1765, -198.6522) (30.4729, -198.6522) (30.7989, -198.215) (30.7989, -197.7753) knots 0 0 0 1 2 2 2
  line L63 (34.1853, -198.9189) -> (34.1853, -197.595)
  spline S79 degree 2 poles (34.1853, -197.595) (34.1853, -197.4369) (34.1606, -197.1677) (34.1211, -197.0936) knots 0 0 0 1 2 2 2
  spline S80 degree 2 poles (34.1211, -197.0936) (34.0816, -197.0121) (33.9309, -196.933) (33.8, -196.933) knots 0 0 0 1 2 2 2
  spline S81 degree 2 poles (33.8, -196.933) (33.6814, -196.933) (33.4097, -197.0788) (33.2665, -197.2171) knots 0 0 0 1 2 2 2
  spline S82 degree 2 poles (33.2665, -197.2171) (33.2689, -197.2517) (33.2739, -197.348) (33.2739, -197.4122) knots 0 0 0 1 2 2 2
  line L64 (33.2739, -197.4122) -> (33.2739, -198.9189)
  line L65 (33.2739, -198.9189) -> (32.8885, -198.9189)
  line L66 (32.8885, -198.9189) -> (32.8885, -197.595)
  spline S83 degree 2 poles (32.8885, -197.595) (32.8885, -197.4369) (32.8638, -197.1677) (32.8243, -197.0936) knots 0 0 0 1 2 2 2
  spline S84 degree 2 poles (32.8243, -197.0936) (32.7848, -197.0121) (32.6341, -196.933) (32.5032, -196.933) knots 0 0 0 1 2 2 2
  spline S85 degree 2 poles (32.5032, -196.933) (32.3797, -196.933) (32.1055, -197.0886) (31.9771, -197.2097) knots 0 0 0 1 2 2 2
  line L67 (31.9771, -197.2097) -> (31.9771, -198.9189)
  line L68 (31.9771, -198.9189) -> (31.5918, -198.9189)
  line L69 (31.5918, -198.9189) -> (31.5918, -196.6317)
  line L70 (31.5918, -196.6317) -> (31.9771, -196.6317)
  line L71 (31.9771, -196.6317) -> (31.9771, -196.8836)
  spline S86 degree 2 poles (31.9771, -196.8836) (32.1278, -196.7329) (32.4242, -196.5675) (32.602, -196.5675) knots 0 0 0 1 2 2 2
  spline S87 degree 2 poles (32.602, -196.5675) (32.8046, -196.5675) (33.1183, -196.7527) (33.1998, -196.9627) knots 0 0 0 1 2 2 2
  spline S88 degree 2 poles (33.1998, -196.9627) (33.3751, -196.7675) (33.7061, -196.5675) (33.8988, -196.5675) knots 0 0 0 1 2 2 2
  spline S89 degree 2 poles (33.8988, -196.5675) (34.047, -196.5675) (34.289, -196.6588) (34.378, -196.7626) knots 0 0 0 1 2 2 2
  spline S90 degree 2 poles (34.378, -196.7626) (34.4694, -196.8663) (34.5706, -197.1776) (34.5706, -197.4122) knots 0 0 0 1 2 2 2
  line L72 (34.5706, -197.4122) -> (34.5706, -198.9189)
  line L73 (34.5706, -198.9189) -> (34.1853, -198.9189)
  spline S91 degree 2 poles (25.9824, -203.0012) (25.9824, -203.2285) (25.8095, -203.5767) (25.6662, -203.6904) knots 0 0 0 1 2 2 2
  spline S92 degree 2 poles (25.6662, -203.6904) (25.4933, -203.8237) (25.1006, -203.9374) (24.7894, -203.9374) knots 0 0 0 1 2 2 2
  line L74 (24.7894, -203.9374) -> (23.915, -203.9374)
  line L75 (23.915, -203.9374) -> (23.915, -200.8894)
  line L76 (23.915, -200.8894) -> (24.7227, -200.8894)
  spline S93 degree 2 poles (24.7227, -200.8894) (25.0487, -200.8894) (25.3748, -200.9314) (25.523, -201.0129) knots 0 0 0 1 2 2 2
  spline S94 degree 2 poles (25.523, -201.0129) (25.6884, -201.0993) (25.8391, -201.3834) (25.8391, -201.576) knots 0 0 0 1 2 2 2
  spline S95 degree 2 poles (25.8391, -201.576) (25.8391, -201.7909) (25.6119, -202.1318) (25.4118, -202.2281) knots 0 0 0 1 2 2 2
  line L77 (25.4118, -202.2281) -> (25.4118, -202.2429)
  spline S96 degree 2 poles (25.4118, -202.2429) (25.6835, -202.317) (25.9824, -202.7098) (25.9824, -203.0012) knots 0 0 0 1 2 2 2
  spline S97 degree 2 poles (25.56, -203.0185) (25.56, -202.8456) (25.4612, -202.6233) (25.313, -202.5443) knots 0 0 0 1 2 2 2
  spline S98 degree 2 poles (25.313, -202.5443) (25.2167, -202.4949) (24.9894, -202.4652) (24.7795, -202.4652) knots 0 0 0 1 2 2 2
  line L78 (24.7795, -202.4652) -> (24.3201, -202.4652)
  line L79 (24.3201, -202.4652) -> (24.3201, -203.5916)
  line L80 (24.3201, -203.5916) -> (24.6486, -203.5916)
  spline S99 degree 2 poles (24.6486, -203.5916) (24.9153, -203.5916) (25.2216, -203.5422) (25.3402, -203.4631) knots 0 0 0 1 2 2 2
  spline S100 degree 2 poles (25.3402, -203.4631) (25.4538, -203.3816) (25.56, -203.1791) (25.56, -203.0185) knots 0 0 0 1 2 2 2
  spline S101 degree 2 poles (25.4167, -201.6328) (25.4167, -201.5242) (25.3426, -201.3611) (25.2611, -201.3142) knots 0 0 0 1 2 2 2
  spline S102 degree 2 poles (25.2611, -201.3142) (25.1623, -201.2599) (24.9227, -201.2352) (24.7078, -201.2352) knots 0 0 0 1 2 2 2
  line L81 (24.7078, -201.2352) -> (24.3201, -201.2352)
  line L82 (24.3201, -201.2352) -> (24.3201, -202.1268)
  line L83 (24.3201, -202.1268) -> (24.7795, -202.1268)
  spline S103 degree 2 poles (24.7795, -202.1268) (24.9697, -202.1268) (25.15, -202.0873) (25.2463, -202.0256) knots 0 0 0 1 2 2 2
  spline S104 degree 2 poles (25.2463, -202.0256) (25.3402, -201.9663) (25.4167, -201.7761) (25.4167, -201.6328) knots 0 0 0 1 2 2 2
  spline S105 degree 2 poles (28.235, -202.7937) (28.235, -203.3717) (27.6793, -204.0016) (27.2149, -204.0016) knots 0 0 0 1 2 2 2
  spline S106 degree 2 poles (27.2149, -204.0016) (26.7382, -204.0016) (26.1923, -203.352) (26.1923, -202.7937) knots 0 0 0 1 2 2 2
  spline S107 degree 2 poles (26.1923, -202.7937) (26.1923, -202.2207) (26.7555, -201.5859) (27.2149, -201.5859) knots 0 0 0 1 2 2 2
  spline S108 degree 2 poles (27.2149, -201.5859) (27.6793, -201.5859) (28.235, -202.2182) (28.235, -202.7937) knots 0 0 0 1 2 2 2
  spline S109 degree 2 poles (27.8374, -202.7937) (27.8374, -202.3491) (27.5138, -201.9169) (27.2149, -201.9169) knots 0 0 0 1 2 2 2
  spline S110 degree 2 poles (27.2149, -201.9169) (26.916, -201.9169) (26.59, -202.3491) (26.59, -202.7937) knots 0 0 0 1 2 2 2
  spline S111 degree 2 poles (26.59, -202.7937) (26.59, -203.226) (26.916, -203.6706) (27.2149, -203.6706) knots 0 0 0 1 2 2 2
  spline S112 degree 2 poles (27.2149, -203.6706) (27.5113, -203.6706) (27.8374, -203.2334) (27.8374, -202.7937) knots 0 0 0 1 2 2 2
  line L84 (30.4062, -203.9374) -> (29.9344, -203.9374)
  line L85 (29.9344, -203.9374) -> (29.3786, -203.0778)
  line L86 (29.3786, -203.0778) -> (28.8081, -203.9374)
  line L87 (28.8081, -203.9374) -> (28.3709, -203.9374)
  line L88 (28.3709, -203.9374) -> (29.1638, -202.8036)
  line L89 (29.1638, -202.8036) -> (28.3783, -201.6501)
  line L90 (28.3783, -201.6501) -> (28.8501, -201.6501)
  line L91 (28.8501, -201.6501) -> (29.4033, -202.5023)
  line L92 (29.4033, -202.5023) -> (29.969, -201.6501)
  line L93 (29.969, -201.6501) -> (30.4062, -201.6501)
  line L94 (30.4062, -201.6501) -> (29.6182, -202.7789)
  line L95 (29.6182, -202.7789) -> (30.4062, -203.9374)
  spline S113 degree 2 poles (31.4708, -201.1784) (31.3596, -201.1784) (31.1398, -201.2327) (31.0336, -201.2747) knots 0 0 0 1 2 2 2
  spline S114 degree 2 poles (31.0336, -201.2747) (30.9348, -201.3167) (30.789, -201.4056) (30.7322, -201.4451) knots 0 0 0 1 2 2 2
  line L96 (30.7322, -201.4451) -> (30.7075, -201.4451)
  line L97 (30.7075, -201.4451) -> (30.7075, -201.0129)
  spline S115 degree 2 poles (30.7075, -201.0129) (30.8409, -200.9412) (31.2979, -200.8251) (31.5029, -200.8251) knots 0 0 0 1 2 2 2
  spline S116 degree 2 poles (31.5029, -200.8251) (31.7103, -200.8251) (32.0191, -200.9091) (32.1451, -200.998) knots 0 0 0 1 2 2 2
  spline S117 degree 2 poles (32.1451, -200.998) (32.2784, -201.0944) (32.4168, -201.3735) (32.4168, -201.5612) knots 0 0 0 1 2 2 2
  spline S118 degree 2 poles (32.4168, -201.5612) (32.4168, -201.8132) (32.0858, -202.1935) (31.8536, -202.2429) knots 0 0 0 1 2 2 2
  line L98 (31.8536, -202.2429) -> (31.8536, -202.2726)
  spline S119 degree 2 poles (31.8536, -202.2726) (31.9499, -202.2923) (32.1698, -202.3813) (32.2636, -202.4702) knots 0 0 0 1 2 2 2
  spline S120 degree 2 poles (32.2636, -202.4702) (32.3575, -202.5566) (32.476, -202.8333) (32.476, -203.0333) knots 0 0 0 1 2 2 2
  spline S121 degree 2 poles (32.476, -203.0333) (32.476, -203.2384) (32.3353, -203.5866) (32.2068, -203.72) knots 0 0 0 1 2 2 2
  spline S122 degree 2 poles (32.2068, -203.72) (32.0734, -203.8583) (31.6955, -204.0016) (31.4559, -204.0016) knots 0 0 0 1 2 2 2
  spline S123 degree 2 poles (31.4559, -204.0016) (31.2262, -204.0016) (30.7767, -203.8904) (30.6235, -203.8139) knots 0 0 0 1 2 2 2
  line L99 (30.6235, -203.8139) -> (30.6235, -203.3816)
  line L100 (30.6235, -203.3816) -> (30.6532, -203.3816)
  spline S124 degree 2 poles (30.6532, -203.3816) (30.7816, -203.4755) (31.2163, -203.6484) (31.4312, -203.6484) knots 0 0 0 1 2 2 2
  spline S125 degree 2 poles (31.4312, -203.6484) (31.5572, -203.6484) (31.8091, -203.5693) (31.8931, -203.4779) knots 0 0 0 1 2 2 2
  spline S126 degree 2 poles (31.8931, -203.4779) (31.9746, -203.3866) (32.0611, -203.1692) (32.0611, -203.0037) knots 0 0 0 1 2 2 2
  spline S127 degree 2 poles (32.0611, -203.0037) (32.0611, -202.8382) (31.9648, -202.6233) (31.8783, -202.5616) knots 0 0 0 1 2 2 2
  spline S128 degree 2 poles (31.8783, -202.5616) (31.7919, -202.4998) (31.5572, -202.4529) (31.4189, -202.4529) knots 0 0 0 1 2 2 2
  line L101 (31.4189, -202.4529) -> (31.246, -202.4529)
  line L102 (31.246, -202.4529) -> (31.246, -202.1145)
  line L103 (31.246, -202.1145) -> (31.3818, -202.1145)
  spline S129 degree 2 poles (31.3818, -202.1145) (31.656, -202.1145) (32.0018, -201.8527) (32.0018, -201.6032) knots 0 0 0 1 2 2 2
  spline S130 degree 2 poles (32.0018, -201.6032) (32.0018, -201.4871) (31.9129, -201.3216) (31.8413, -201.2722) knots 0 0 0 1 2 2 2
  spline S131 degree 2 poles (31.8413, -201.2722) (31.7647, -201.2203) (31.577, -201.1784) (31.4708, -201.1784) knots 0 0 0 1 2 2 2
  spline S132 degree 2 poles (20.6212, -207.9876) (20.6212, -208.2074) (20.4804, -208.5828) (20.352, -208.7212) knots 0 0 0 1 2 2 2
  spline S133 degree 2 poles (20.352, -208.7212) (20.2235, -208.8595) (19.8407, -209.02) (19.6036, -209.02) knots 0 0 0 1 2 2 2
  spline S134 degree 2 poles (19.6036, -209.02) (19.3862, -209.02) (18.9614, -208.9237) (18.8057, -208.8471) knots 0 0 0 1 2 2 2
  line L104 (18.8057, -208.8471) -> (18.8057, -208.4149)
  line L105 (18.8057, -208.4149) -> (18.8354, -208.4149)
  spline S135 degree 2 poles (18.8354, -208.4149) (18.8823, -208.4495) (19.0577, -208.5384) (19.1639, -208.5779) knots 0 0 0 1 2 2 2
  spline S136 degree 2 poles (19.1639, -208.5779) (19.2849, -208.6199) (19.485, -208.6668) (19.611, -208.6668) knots 0 0 0 1 2 2 2
  spline S137 degree 2 poles (19.611, -208.6668) (19.7345, -208.6668) (19.9667, -208.5779) (20.0506, -208.4816) knots 0 0 0 1 2 2 2
  spline S138 degree 2 poles (20.0506, -208.4816) (20.1272, -208.3902) (20.2062, -208.1481) (20.2062, -207.9851) knots 0 0 0 1 2 2 2
  spline S139 degree 2 poles (20.2062, -207.9851) (20.2062, -207.8221) (20.1173, -207.6146) (20.0333, -207.5454) knots 0 0 0 1 2 2 2
  spline S140 degree 2 poles (20.0333, -207.5454) (19.9469, -207.4689) (19.69, -207.4046) (19.5344, -207.4046) knots 0 0 0 1 2 2 2
  spline S141 degree 2 poles (19.5344, -207.4046) (19.3664, -207.4046) (19.033, -207.4565) (18.9317, -207.4787) knots 0 0 0 1 2 2 2
  line L106 (18.9317, -207.4787) -> (18.9317, -205.9078)
  line L107 (18.9317, -205.9078) -> (20.6039, -205.9078)
  line L108 (20.6039, -205.9078) -> (20.6039, -206.266)
  line L109 (20.6039, -206.266) -> (19.3244, -206.266)
  line L110 (19.3244, -206.266) -> (19.3244, -207.0786)
  spline S142 degree 2 poles (19.3244, -207.0786) (19.3985, -207.0687) (19.5418, -207.0613) (19.6011, -207.0613) knots 0 0 0 1 2 2 2
  spline S143 degree 2 poles (19.6011, -207.0613) (19.8357, -207.0613) (20.1593, -207.1379) (20.3075, -207.2515) knots 0 0 0 1 2 2 2
  spline S144 degree 2 poles (20.3075, -207.2515) (20.4582, -207.3651) (20.6212, -207.7109) (20.6212, -207.9876) knots 0 0 0 1 2 2 2
  line L111 (22.328, -205.772) -> (21.135, -209.6178)
  line L112 (21.135, -209.6178) -> (20.7892, -209.6178)
  line L113 (20.7892, -209.6178) -> (21.9772, -205.772)
  line L114 (21.9772, -205.772) -> (22.328, -205.772)
  line L115 (24.5436, -208.9558) -> (22.6639, -208.9558)
  line L116 (22.6639, -208.9558) -> (22.6639, -208.5236)
  spline S145 degree 2 poles (22.6639, -208.5236) (22.8665, -208.3334) (23.2271, -207.9802) (23.4, -207.79) knots 0 0 0 1 2 2 2
  spline S146 degree 2 poles (23.4, -207.79) (23.7482, -207.4071) (24.0027, -206.9477) (24.0027, -206.7032) knots 0 0 0 1 2 2 2
  spline S147 degree 2 poles (24.0027, -206.7032) (24.0027, -206.5747) (23.9236, -206.3821) (23.852, -206.3203) knots 0 0 0 1 2 2 2
  spline S148 degree 2 poles (23.852, -206.3203) (23.7804, -206.2586) (23.5926, -206.1968) (23.479, -206.1968) knots 0 0 0 1 2 2 2
  spline S149 degree 2 poles (23.479, -206.1968) (23.3703, -206.1968) (23.148, -206.2512) (23.0468, -206.2931) knots 0 0 0 1 2 2 2
  spline S150 degree 2 poles (23.0468, -206.2931) (22.9603, -206.3277) (22.7998, -206.4265) (22.7504, -206.4611) knots 0 0 0 1 2 2 2
  line L117 (22.7504, -206.4611) -> (22.7281, -206.4611)
  line L118 (22.7281, -206.4611) -> (22.7281, -206.0264)
  spline S151 degree 2 poles (22.7281, -206.0264) (22.8541, -205.9646) (23.3061, -205.8436) (23.5087, -205.8436) knots 0 0 0 1 2 2 2
  spline S152 degree 2 poles (23.5087, -205.8436) (23.936, -205.8436) (24.4176, -206.2956) (24.4176, -206.6809) knots 0 0 0 1 2 2 2
  spline S153 degree 2 poles (24.4176, -206.6809) (24.4176, -206.8612) (24.3336, -207.1626) (24.2595, -207.291) knots 0 0 0 1 2 2 2
  spline S154 degree 2 poles (24.2595, -207.291) (24.1854, -207.4244) (23.9705, -207.6862) (23.852, -207.8122) knots 0 0 0 1 2 2 2
  spline S155 degree 2 poles (23.852, -207.8122) (23.6593, -208.0222) (23.1876, -208.4717) (23.0468, -208.6026) knots 0 0 0 1 2 2 2
  line L119 (23.0468, -208.6026) -> (24.5436, -208.6026)
  line L120 (24.5436, -208.6026) -> (24.5436, -208.9558)
  line L121 (26.8308, -208.9558) -> (24.9511, -208.9558)
  line L122 (24.9511, -208.9558) -> (24.9511, -208.5236)
  spline S156 degree 2 poles (24.9511, -208.5236) (25.1537, -208.3334) (25.5143, -207.9802) (25.6872, -207.79) knots 0 0 0 1 2 2 2
  spline S157 degree 2 poles (25.6872, -207.79) (26.0355, -207.4071) (26.2899, -206.9477) (26.2899, -206.7032) knots 0 0 0 1 2 2 2
  spline S158 degree 2 poles (26.2899, -206.7032) (26.2899, -206.5747) (26.2109, -206.3821) (26.1392, -206.3203) knots 0 0 0 1 2 2 2
  spline S159 degree 2 poles (26.1392, -206.3203) (26.0676, -206.2586) (25.8799, -206.1968) (25.7662, -206.1968) knots 0 0 0 1 2 2 2
  spline S160 degree 2 poles (25.7662, -206.1968) (25.6576, -206.1968) (25.4353, -206.2512) (25.334, -206.2931) knots 0 0 0 1 2 2 2
  spline S161 degree 2 poles (25.334, -206.2931) (25.2475, -206.3277) (25.087, -206.4265) (25.0376, -206.4611) knots 0 0 0 1 2 2 2
  line L123 (25.0376, -206.4611) -> (25.0154, -206.4611)
  line L124 (25.0154, -206.4611) -> (25.0154, -206.0264)
  spline S162 degree 2 poles (25.0154, -206.0264) (25.1413, -205.9646) (25.5933, -205.8436) (25.7959, -205.8436) knots 0 0 0 1 2 2 2
  spline S163 degree 2 poles (25.7959, -205.8436) (26.2232, -205.8436) (26.7049, -206.2956) (26.7049, -206.6809) knots 0 0 0 1 2 2 2
  spline S164 degree 2 poles (26.7049, -206.6809) (26.7049, -206.8612) (26.6209, -207.1626) (26.5468, -207.291) knots 0 0 0 1 2 2 2
  spline S165 degree 2 poles (26.5468, -207.291) (26.4727, -207.4244) (26.2578, -207.6862) (26.1392, -207.8122) knots 0 0 0 1 2 2 2
  spline S166 degree 2 poles (26.1392, -207.8122) (25.9466, -208.0222) (25.4748, -208.4717) (25.334, -208.6026) knots 0 0 0 1 2 2 2
  line L125 (25.334, -208.6026) -> (26.8308, -208.6026)
  line L126 (26.8308, -208.6026) -> (26.8308, -208.9558)
  line L127 (28.5055, -205.772) -> (27.3125, -209.6178)
  line L128 (27.3125, -209.6178) -> (26.9667, -209.6178)
  line L129 (26.9667, -209.6178) -> (28.1548, -205.772)
  line L130 (28.1548, -205.772) -> (28.5055, -205.772)
  line L131 (30.7211, -208.9558) -> (28.8414, -208.9558)
  line L132 (28.8414, -208.9558) -> (28.8414, -208.5236)
  spline S167 degree 2 poles (28.8414, -208.5236) (29.044, -208.3334) (29.4046, -207.9802) (29.5775, -207.79) knots 0 0 0 1 2 2 2
  spline S168 degree 2 poles (29.5775, -207.79) (29.9258, -207.4071) (30.1802, -206.9477) (30.1802, -206.7032) knots 0 0 0 1 2 2 2
  spline S169 degree 2 poles (30.1802, -206.7032) (30.1802, -206.5747) (30.1011, -206.3821) (30.0295, -206.3203) knots 0 0 0 1 2 2 2
  spline S170 degree 2 poles (30.0295, -206.3203) (29.9579, -206.2586) (29.7701, -206.1968) (29.6565, -206.1968) knots 0 0 0 1 2 2 2
  spline S171 degree 2 poles (29.6565, -206.1968) (29.5478, -206.1968) (29.3255, -206.2512) (29.2243, -206.2931) knots 0 0 0 1 2 2 2
  spline S172 degree 2 poles (29.2243, -206.2931) (29.1378, -206.3277) (28.9773, -206.4265) (28.9279, -206.4611) knots 0 0 0 1 2 2 2
  line L133 (28.9279, -206.4611) -> (28.9056, -206.4611)
  line L134 (28.9056, -206.4611) -> (28.9056, -206.0264)
  spline S173 degree 2 poles (28.9056, -206.0264) (29.0316, -205.9646) (29.4836, -205.8436) (29.6862, -205.8436) knots 0 0 0 1 2 2 2
  spline S174 degree 2 poles (29.6862, -205.8436) (30.1135, -205.8436) (30.5951, -206.2956) (30.5951, -206.6809) knots 0 0 0 1 2 2 2
  spline S175 degree 2 poles (30.5951, -206.6809) (30.5951, -206.8612) (30.5112, -207.1626) (30.4371, -207.291) knots 0 0 0 1 2 2 2
  spline S176 degree 2 poles (30.4371, -207.291) (30.3629, -207.4244) (30.1481, -207.6862) (30.0295, -207.8122) knots 0 0 0 1 2 2 2
  spline S177 degree 2 poles (30.0295, -207.8122) (29.8368, -208.0222) (29.3651, -208.4717) (29.2243, -208.6026) knots 0 0 0 1 2 2 2
  line L135 (29.2243, -208.6026) -> (30.7211, -208.6026)
  line L136 (30.7211, -208.6026) -> (30.7211, -208.9558)
  spline S178 degree 2 poles (33.0256, -207.4318) (33.0256, -208.2519) (32.5489, -209.02) (32.0524, -209.02) knots 0 0 0 1 2 2 2
  spline S179 degree 2 poles (32.0524, -209.02) (31.5486, -209.02) (31.0768, -208.237) (31.0768, -207.4343) knots 0 0 0 1 2 2 2
  spline S180 degree 2 poles (31.0768, -207.4343) (31.0768, -206.6093) (31.5535, -205.8461) (32.0524, -205.8461) knots 0 0 0 1 2 2 2
  spline S181 degree 2 poles (32.0524, -205.8461) (32.5539, -205.8461) (33.0256, -206.6365) (33.0256, -207.4318) knots 0 0 0 1 2 2 2